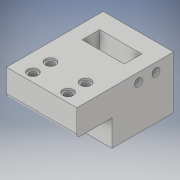
# Autodesk Inventor part: Swivel Joint Driver
Saved by Autodesk Inventor 2019 (Build 230136000, 136)
## iProperties
Created: 2020-04-05
Part Number: Swivel Joint Driver
Material: Generic
Document SubType Name: Modeling
Designer: isaac
Density: 1 g/cm^3
Appearance: Default
Author: isaac
Autodesk Inventor part; units mm, degrees
ref_plane "YZ Plane" through (0, 0, 0) normal (1, 0, 0) x (0, 1, 0)
ref_plane "XZ Plane" through (0, 0, 0) normal (0, 1, 0) x (-1, 0, 0)
ref_plane "XY Plane" through (0, 0, 0) normal (0, 0, 1) x (1, 0, 0)
sketch "Sketch1" plane through (0, 0, 0) normal (0, 1, 0) x (-1, 0, 0)
  line L0 (-20, 10) -> (20, 10)
  line L1 (20, 10) -> (20, -10)
  line L2 (20, -10) -> (-20, -10)
  line L3 (-20, -10) -> (-20, 10)
  line L4 (-20, 10) -> (20, -10) construction
  line L5 (20, 10) -> (-20, -10) construction
  point P0 (0, 0)
  dimension "d0" = 40
  dimension "d1" = 20
  constraints: 12 end point, 2 midpoint, 2 parallel, 1 horizontal, 1 perpendicular
  measures "d0" distance of L1.end L2.end
  measures "d1" distance of L0.end L1.end
extrude "Extrusion1" add sketch "Sketch1" along normal blind 15
sketch "Sketch2" plane through (0, 15, 0) normal (0, 1, 0) x (1, 0, 0)
  line L0 (20, 10) -> (-20, 10) construction
  line L1 (-20, -10) -> (20, -10) construction
  line L2 (20, -10) -> (20, 10) construction
  line L3 (20, 10) -> (-20, 10) construction
  line L4 (-20, 10) -> (-20, -10) construction
  line L5 (-20, -10) -> (20, 10) construction
  line L6 (20, -10) -> (-20, 10) construction
  line L7 (-10, -5) -> (10, -5) construction
  line L8 (10, -5) -> (10, 5) construction
  line L9 (10, 5) -> (-10, 5) construction
  line L10 (-10, 5) -> (-10, -5) construction
  line L11 (-10, -5) -> (10, 5) construction
  line L12 (10, -5) -> (-10, 5) construction
  point P0 (0, 0)
  dimension "d4" = 20
  constraints: 24 end point, 4 coincident, 4 midpoint, 4 parallel, 2 horizontal, 2 perpendicular, 1 point on line
  measures "d4" distance of L9.end L8.end
hole "Hole1" at (-10, 15, -5) at (-10, 15, 5) at (10, 15, 5) at (10, 15, -5) direction (0, -1, 0) diameter 4 end through all counterbore diameter 6 counterbore depth 1
fillet "Fillet1" radius 2 1 edges at (0, 0, 10)
sketch "Sketch3" plane through (20, 0, -10) normal (1, 0, 0) x (0, 0, -1)
  line L0 (0, 0) -> (0, 15) projected
  line L1 (0, 15) -> (5, 15)
  line L2 (5, 15) -> (5, -15)
  line L3 (5, -15) -> (0, -15)
  line L4 (0, -15) -> (0, 15)
  point P0 (-10, 0)
  dimension "d13" = 5
  dimension "d14" = 30
  constraints: 8 end point, 2 parallel, 1 horizontal, 1 perpendicular
  measures "d13" distance of L2.end L3.end
  measures "d14" distance of L1.end L2.end
extrude "Extrusion2" add sketch "Sketch3" against normal up to surface (40 mm away)
sketch "Sketch4" plane through (20, -15, -15) normal (0, 0, -1) x (-1, 0, 0)
  line L0 (0, 17) -> (0, 30) projected
  line L1 (0, 0) -> (40, 0) projected
  line L2 (0, 30) -> (40, 30)
  line L3 (40, 30) -> (40, 0)
  line L4 (40, 0) -> (0, 0)
  line L5 (0, 0) -> (0, 30)
  point P0 (20, 15)
  constraints: 8 end point, 2 parallel, 1 horizontal, 1 perpendicular
extrude "Extrusion3" add sketch "Sketch4" along normal blind 10
sketch "Sketch5" plane through (20, -15, -25) normal (0, 0, -1) x (-1, 0, 0)
  point P0 (20, 15)
  point P1 (20, 15)
  constraints: 1 coincident
hole "Hole2" at (0, 0, -25) direction (0, 0, 1) diameter 7.5 depth 10
sketch "Sketch6" plane through (20, -15, -25) normal (0, 0, -1) x (-1, 0, 0)
  point P0 (20, 15)
  point P1 (20, 15)
  constraints: 1 coincident
hole "Hole3" at (0, 0, -25) direction (0, 0, 1) diameter 20 depth 6.5
sketch "Sketch7" plane through (20, -15, -25) normal (0, 0, -1) x (-1, 0, 0)
  line L0 (40, 0) -> (40, 30) projected
  line L1 (40, 30) -> (0, 30) projected
  line L2 (40, 0) -> (32, 0)
  line L3 (32, 0) -> (32, 30)
  line L4 (32, 30) -> (40, 30)
  line L5 (40, 30) -> (40, 0)
  line L6 (0, 0) -> (40, 0) construction
  line L7 (20, 0) -> (20, 30) construction
  line L8 (0, 0) -> (0, 30)
  line L9 (0, 0) -> (8, 0)
  line L10 (8, 0) -> (8, 30)
  line L11 (8, 30) -> (0, 30)
  line L12 (0, 30) -> (0, 0)
  point P0 (20, 15)
  dimension "d33" = 8
  constraints: 20 end point, 4 symmetric about line, 2 midpoint, 2 parallel, 1 horizontal, 1 perpendicular, 1 point on line
  measures "d33" distance of L3.end L4.end
extrude "Extrusion4" add sketch "Sketch7" along normal blind 10
sketch "Sketch8" plane through (20, -15, -35) normal (0, 0, -1) x (-1, 0, 0)
  line L0 (40, 15) -> (40, 0) projected
  line L1 (40, 30) -> (0, 30) projected
  line L2 (40, 0) -> (0, 0)
  line L3 (0, 0) -> (0, 30)
  line L4 (0, 30) -> (40, 30)
  line L5 (40, 30) -> (40, 0)
  point P0 (20, 15)
  constraints: 8 end point, 2 parallel, 1 horizontal, 1 perpendicular
extrude "Extrusion5" add sketch "Sketch8" along normal blind 10
sketch "Sketch9" plane through (20, -15, -45) normal (0, 0, -1) x (-1, 0, 0)
  line L0 (40, 15) -> (40, 0) construction
  line L1 (0, 17) -> (0, 30) construction
  line L2 (40, 0) -> (0, 30) construction
  line L3 (40, 17) -> (40, 30) construction
  line L4 (0, 0) -> (0, 15) construction
  line L5 (40, 30) -> (0, 0) construction
  point P0 (20, 15)
  point P1 (20, 15)
  constraints: 4 end point, 1 coincident
hole "Hole4" at (0, 0, -45) direction (0, 0, 1) diameter 7.5 depth 10 counterbore diameter 19.5 counterbore depth 6
sketch "Sketch10" plane through (-20, 2, 10) normal (-1, 0, 0) x (0, 0, 1)
  line L0 (-55, -17) -> (-55, 13) construction
  line L1 (-55, 13) -> (-45, 13) construction
  line L2 (-45, 13) -> (-45, 8) construction
  line L3 (-45, 8) -> (-55, 8) construction
  line L4 (-55, 8) -> (-55, 13) construction
  line L5 (-55, 13) -> (-35, 13) construction
  line L6 (-35, 13) -> (-35, 8) construction
  line L7 (-35, 8) -> (-55, 8) construction
  line L8 (-55, 8) -> (-55, 13) construction
  point P0 (-10, -2)
  dimension "d45" = 10
  dimension "d46" = 5
  dimension "d47" = 20
  constraints: 16 end point, 4 parallel, 2 coincident, 2 horizontal, 2 perpendicular
  measures "d45" distance of L2.end L3.end
  measures "d46" distance of L1.end L2.end
  measures "d47" distance of L6.end L7.end
hole "Hole5" at (-20, 10, -35) at (-20, 10, -25) direction (1, 0, 0) diameter 3.5 depth 7 counterbore diameter 4.5 counterbore depth 6
mirror "Mirror1" about plane through (0, 0, 0) normal (1, 0, 0) of "Hole5"
body "Solid1"
